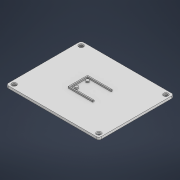
# Autodesk Inventor part: BH1750-viko
Saved by Autodesk Inventor 2022 (Build 260153000, 153)
## iProperties
Created: 2023-05-13
Part Number: BH1750-viko
Material: Všeobecné
Document SubType Name: Modeling
Designer: tada
Density: 1 g/cm^3
Appearance: Výchozí
Author: tada
Autodesk Inventor part; units mm, degrees
ref_plane "YZ Plane" through (0, 0, 0) normal (1, 0, 0) x (0, 1, 0)
ref_plane "XZ Plane" through (0, 0, 0) normal (0, 1, 0) x (-1, 0, 0)
ref_plane "XY Plane" through (0, 0, 0) normal (0, 0, 1) x (1, 0, 0)
sketch "Náčrt1" plane through (0, 0, 0) normal (0, 1, 0) x (-1, 0, 0)
  line L0 (0, 0) -> (-75, 0)
  line L1 (-75, 0) -> (-75, -60)
  line L2 (-75, -60) -> (0, -60)
  line L3 (0, -60) -> (0, 0)
  line L4 (2, 2) -> (-77, 2)
  line L5 (-77, 2) -> (-77, -62)
  line L6 (-77, -62) -> (2, -62)
  line L7 (2, -62) -> (2, 2)
  dimension "d0" = 2
  dimension "d1" = 2
  dimension "d2" = 2
  dimension "d3" = 2
  dimension "d4" = 75
  dimension "d5" = 60
  constraints: 16 end point, 4 parallel, 2 horizontal, 2 perpendicular
  measures "d0" distance between parallel lines of L7 L3
  measures "d1" distance between parallel lines of L6 L2
  measures "d2" distance between parallel lines of L1 L5
  measures "d3" distance between parallel lines of L0 L4
  measures "d4" distance of L1.end L2.end
  measures "d5" distance of L0.end L1.end
extrude "Vysunutí1" add sketch "Náčrt1" along normal blind 2 contours L3 L2 L1 L0 | L7 L6 L5 L4
sketch "Náčrt2" plane through (0, 2, 0) normal (0, 1, 0) x (1, 0, 0)
  circle A0 centre (1.5, 1.5) radius 1.5
  circle A1 centre (1.5, 58.5) radius 1.5
  circle A2 centre (73.5, 58.5) radius 1.5
  circle A3 centre (73.5, 1.5) radius 1.5
  line L0 (-2, 62) -> (-2, -2) projected
  line L1 (-2, -2) -> (77, -2) projected
  line L2 (77, 62) -> (-2, 62) projected
  line L3 (77, -2) -> (77, 62) projected
  point P0 (0, 0)
  dimension "d8" = 3
  dimension "d9" = 3
  dimension "d10" = 3
  dimension "d11" = 3
  dimension "d12" = 3.5
  dimension "d13" = 3.5
  dimension "d14" = 3.5
  dimension "d15" = 3.5
  dimension "d16" = 3.5
  dimension "d17" = 3.5
  dimension "d18" = 3.5
  dimension "d19" = 3.5
  constraints: 4 centre point
  measures "d8" diameter of A0
  measures "d9" diameter of A3
  measures "d10" diameter of A2
  measures "d11" diameter of A1
  measures "d12" distance from line of L0 A0.centre
  measures "d13" distance from line of L1 A0.centre
  measures "d14" distance from line of L0 A1.centre
  measures "d15" distance from line of L2 A1.centre
  measures "d16" distance from line of L2 A2.centre
  measures "d17" distance from line of A2.centre L3
  measures "d18" distance from line of L1 A3.centre
  measures "d19" distance from line of A3.centre L3
extrude "Vysunutí2" cut sketch "Náčrt2" against normal blind 2 contours A0 | A1 | A2 | A3
chamfer "Zkosení1" distance 0.5 angle 45 4 edges at (0, 2, -1.5) (0, 2, -58.5) (72, 2, -58.5) (72, 2, -1.5)
fillet "Zaoblení1" radius 2 4 edges at (77, 1, 2) (77, 1, -62) (-2, 1, -62) (-2, 1, 2)
sketch "Náčrt3" plane through (0, 2, 0) normal (0, 1, 0) x (1, 0, 0)
  line L0 (28.2, 22.75) -> (47.2, 22.75)
  line L1 (47.2, 22.75) -> (47.2, 37.25)
  line L2 (47.2, 37.25) -> (28.2, 37.25)
  line L3 (28.2, 37.25) -> (28.2, 22.75)
  circle A0 centre (30.75, 25.3) radius 1.35
  circle A1 centre (30.75, 34.7) radius 1.35
  line L4 (0, -2) -> (75, -2) projected
  line L5 (-2, 60) -> (-2, 0) projected
  line L6 (77, 0) -> (77, 60) projected
  line L7 (27.2, 21.75) -> (48.2, 21.75)
  line L8 (48.2, 21.75) -> (48.2, 38.25)
  line L9 (48.2, 38.25) -> (27.2, 38.25)
  line L10 (27.2, 38.25) -> (27.2, 21.75)
  point P0 (0, 0)
  dimension "d26" = 14.5
  dimension "d27" = 19
  dimension "d28" = 2.55
  dimension "d29" = 2.7
  dimension "d30" = 2.55
  dimension "d31" = 2.7
  dimension "d32" = 2.55
  dimension "d33" = 2.55
  dimension "d34" = 24.75
  dimension "d35" = 30.2
  dimension "d36" = 79
  dimension "d37" = 1
  dimension "d38" = 1
  dimension "d39" = 1
  dimension "d40" = 1
  dimension "d47" = 9.4
  constraints: 16 end point, 4 parallel, 2 centre point, 2 horizontal, 2 perpendicular
  measures "d26" distance between parallel lines of L0 L2
  measures "d27" distance of L1.end L2.end
  measures "d28" distance from line of L0 A0.centre
  measures "d29" diameter of A0
  measures "d30" distance from line of L3 A0.centre
  measures "d31" diameter of A1
  measures "d32" distance from line of L3 A1.centre
  measures "d33" distance from line of L2 A1.centre
  measures "d34" distance between parallel lines of L4 L0
  measures "d35" distance between parallel lines of L5 L3
  measures "d36" distance between parallel lines of L6 L5
  measures "d37" distance between parallel lines of L10 L3
  measures "d38" distance between parallel lines of L7 L0
  measures "d39" distance between parallel lines of L2 L9
  measures "d40" distance between parallel lines of L1 L8
  measures "d47" distance of A0.centre A1.centre
extrude "Vysunutí3" add sketch "Náčrt3" along normal blind 1.2 contours L10 L9 L8 L7
extrude "Vysunutí4" add sketch "Náčrt3" along normal blind 1.2 contours A0 | A1
sketch "Náčrt4" plane through (48.2, 2, -21.75) normal (1, 0, 0) x (0, 0, -1)
  line L0 (1, 0) -> (1, 1.2) projected
  line L1 (15.5, 0) -> (15.5, 1.2) projected
  line L2 (1, 1.2) -> (15.5, 1.2)
  line L3 (15.5, 1.2) -> (15.5, 0)
  line L4 (15.5, 0) -> (1, 0)
  line L5 (1, 0) -> (1, 1.2)
  point P0 (-21.75, -2)
  constraints: 8 end point, 2 parallel, 1 horizontal, 1 perpendicular
extrude "Vysunutí5" cut sketch "Náčrt4" against normal blind 1.2
equation "\"d1\" = d0"
equation "\"d2\" = d0"
equation "\"d3\" = d0"
equation "\"d9\" = d8"
equation "\"d10\" = d8"
equation "\"d11\" = d8"
equation "\"d14\" = d12"
equation "\"d15\" = d12"
equation "\"d16\" = d12"
equation "\"d17\" = d12"
equation "\"d18\" = d12"
equation "\"d19\" = d12"
equation "\"d32\" = d30"
equation "\"d33\" = d28"
equation "\"d38\" = d37"
equation "\"d39\" = d37"
equation "\"d40\" = d37"
